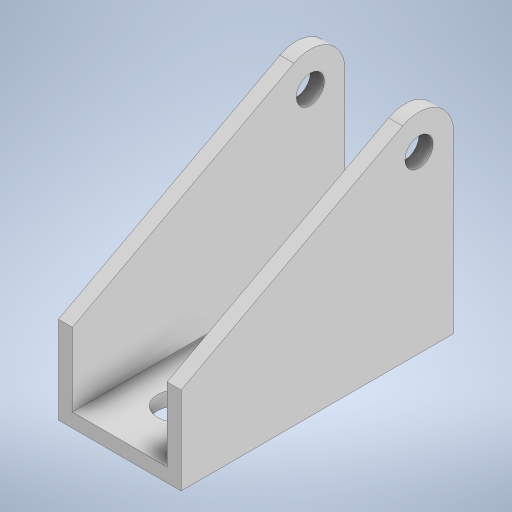
# Autodesk Inventor part: 높이액추브라켓
Saved by Autodesk Inventor 2024 (Build 280153000, 153)
## iProperties
Created: 2024-04-12
Part Number: 높이액추브라켓
Material: 일반
Document SubType Name: Modeling
Designer: kkamin5
Density: 1 g/cm^3
Appearance: 기본값
Author: kkamin5
Autodesk Inventor part; units mm, degrees
ref_plane "YZ Plane" through (0, 0, 0) normal (1, 0, 0) x (0, 1, 0)
ref_plane "XZ Plane" through (0, 0, 0) normal (0, 1, 0) x (-1, 0, 0)
ref_plane "XY Plane" through (0, 0, 0) normal (0, 0, 1) x (1, 0, 0)
sketch "스케치1" plane through (0, 0, 0) normal (1, 0, 0) x (0, 1, 0)
  line L0 (0, 0) -> (0, 58.2)
  line L1 (0, 58.2) -> (18.65, 58.2)
  line L2 (0, 0) -> (37.3, 0)
  circle A0 centre (37.3, 7.4) radius 7.4
  circle A1 centre (37.3, 7.4) radius 3
  line L3 (18.65, 58.2) -> (43.8327, 10.8763)
  dimension "d3" = 14.8
  dimension "d0" = 58.2
  dimension "d1" = 37.3
  dimension "d2" = 18.65
  dimension "d4" = 0
  dimension "d5" = 6
  constraints: 8 end point, 3 horizontal, 1 centre point, 1 coincident, 1 vertical, 4 other
  measures "d0" distance of L0.start L0.end
  measures "d1" distance of L0.start L2.end
  measures "d2" distance of L0.end L1.end
  measures "d4" horizontal distance of point (37.3, 7.4) L2.end
  measures "d5" diameter of A1
extrude "돌출1" add sketch "스케치1" along normal mid plane 26.2
sketch "스케치2" plane through (-13.1, 0, 58.2) normal (0, 0, 1) x (1, 0, 0)
  line L0 (3, 3) -> (23.2, 3)
  line L1 (23.2, 3) -> (23.2, 55.8283)
  line L2 (23.2, 55.8283) -> (3, 55.8283)
  line L3 (3, 55.8283) -> (3, 3)
  line L4 (26.2, 43.8327) -> (26.2, 18.65) projected
  line L5 (26.2, 0) -> (0, 0) projected
  line L6 (0, 18.65) -> (0, 43.8327) projected
  point P0 (13.1, 0)
  dimension "d8" = 3
  dimension "d9" = 3
  dimension "d10" = 3
  constraints: 8 end point, 2 parallel, 1 horizontal, 1 perpendicular
  measures "d8" distance between parallel lines of L4 L1
  measures "d9" distance between parallel lines of L5 L0
  measures "d10" distance between parallel lines of L6 L3
extrude "돌출2" cut sketch "스케치2" against normal through all
sketch "스케치3" plane through (-10.1, 3, 58.2) normal (0, 1, 0) x (1, 0, 0)
  circle A0 centre (10.1, 48.6) radius 4.5
  line L0 (0, 58.2) -> (20.2, 58.2) projected
  line L1 (14.6, 58.2) -> (5.6, 58.2)
  line L2 (5.6, 58.2) -> (5.6, 48.6)
  line L3 (5.6, 48.6) -> (14.6, 48.6)
  line L4 (14.6, 48.6) -> (14.6, 58.2)
  circle A1 centre (10.1, 12.3112) radius 4.25
  point P0 (10.1, 58.2)
  point P1 (10.1, 58.2)
  point P2 (10.1, 48.6)
  point P3 (10.1, 58.2)
  point P4 (14.6, 48.6)
  dimension "d13" = 9
  dimension "d14" = 9
  dimension "d15" = 9.6
  dimension "d16" = 0
  dimension "d17" = 8.5
  dimension "d18" = 0
  constraints: 8 end point, 4 midpoint, 2 parallel, 1 centre point, 1 horizontal, 1 perpendicular, 1 point on line, 3 other
  measures "d14" distance of L2.end L3.end
  measures "d15" distance of L3.end L1.start
  measures "d16" horizontal distance of point (10.1, 58.2) point (10.1, 48.6)
  measures "d17" diameter of A1
  measures "d18" horizontal distance of A1.centre point (10.1, 58.2)
extrude "돌출3" cut sketch "스케치3" against normal through all
equation "\"d2\" = 0.5 * d1"
